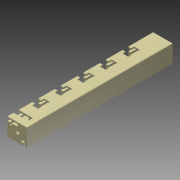
# Autodesk Inventor part: Pillar
Saved by Autodesk Inventor 2015 (Build 190159000, 159)
## iProperties
Created: 2015-04-20
Part Number: Pillar
Material: NylonD2W
Document SubType Name: Modeling
Designer: Akovo_000
Density: 1.13 g/cm^3
Appearance: Nylon 6
Mass: 42.2075 g
Surface Area: 197.531 cm^2
Volume: 37.3518 cm^3
Author: Akovo_000
Autodesk Inventor part; units mm, degrees
ref_plane "YZ Plane" through (0, 0, 0) normal (1, 0, 0) x (0, 1, 0)
ref_plane "XZ Plane" through (0, 0, 0) normal (0, 1, 0) x (-1, 0, 0)
ref_plane "XY Plane" through (0, 0, 0) normal (0, 0, 1) x (1, 0, 0)
sketch "Sketch1" plane through (0, 0, 0) normal (0, 1, 0) x (-1, 0, 0)
  line L0 (20, 18) -> (0, 18)
  line L1 (0, 18) -> (0, 0)
  line L2 (20, 18) -> (20, 16.5)
  line L3 (20, 16.5) -> (15.5, 16.5)
  line L4 (20, 14) -> (20, 0)
  line L5 (0, 0) -> (1.5, 0)
  line L6 (1.5, 0) -> (1.5, 4.5)
  line L7 (1.5, 4.5) -> (4, 4.5)
  line L8 (4, 0) -> (20, 0)
  circle A0 centre (10, 9) radius 2
  line L9 (15.5, 12) -> (17.5, 12)
  line L10 (17.5, 12) -> (17.5, 14)
  line L11 (17.5, 14) -> (20, 14)
  line L12 (15.5, 12) -> (15.5, 14)
  line L13 (4, 0) -> (4, 2.5)
  line L14 (4, 2.5) -> (6, 2.5)
  line L15 (6, 2.5) -> (6, 4.5)
  line L16 (4, 4.5) -> (6, 4.5)
  line L17 (10, 9) -> (0, 9) construction
  line L18 (10, 9) -> (20, 9) construction
  line L19 (10, 9) -> (10, 18) construction
  line L20 (10, 9) -> (10, 0) construction
  line L21 (15.5, 16.5) -> (9.5, 16.5)
  line L22 (9.5, 16.5) -> (9.5, 14)
  line L23 (15.5, 14) -> (9.5, 14)
  dimension "d0" = 2.5
  dimension "d2" = 20
  dimension "d3" = 1.5
  dimension "d7" = 4
  dimension "d13" = 2
  dimension "d26" = 18
  dimension "d84" = 4.5
  dimension "d85" = 4.5
  dimension "d86" = 6
  constraints: 48 end point, 8 equal length, 8 perpendicular, 7 horizontal, 5 point on line, 4 vertical, 2 collinear, 2 midpoint, 1 centre point, 1 parallel
  measures "d0" distance of L2.end L4.start
  measures "d2" distance between parallel lines of L1 L2
  measures "d3" distance between parallel lines of L3 L0
  measures "d7" diameter of A0
  measures "d13" distance of L9.start L12.end
  measures "d26" distance of L0.end L1.end
  measures "d84" distance of L5.end L6.end
  measures "d85" distance of L3.end L2.end
  measures "d86" distance of L21.end L3.end
extrude "Attachment Bas" add sketch "Sketch1" along normal blind 6.5
sketch "Sketch2" plane through (0, 6.5, 0) normal (0, 1, 0) x (1, 0, 0)
  circle A0 centre (-10, -9) radius 2 projected
  line L0 (-13.004, -6.2964) -> (-9.1606, -5.0467)
  line L1 (-9.1606, -5.0467) -> (-6.1566, -7.7503)
  line L2 (-6.1566, -7.7503) -> (-6.996, -11.7036)
  line L3 (-6.996, -11.7036) -> (-10.8394, -12.9533)
  line L4 (-10.8394, -12.9533) -> (-13.8434, -10.2497)
  line L5 (-13.8434, -10.2497) -> (-13.004, -6.2964)
  line L6 (-20, 0) -> (-13.004, -6.2964) construction
  line L7 (-13.004, -6.2964) -> (-10, -9) construction
  line L8 (0, -18) -> (-10, -9) construction
  dimension "d21" = 7
  constraints: 18 end point, 1 coincident, 1 collinear, 13 other
  measures "d21" distance between parallel lines of L1 L4
extrude "BossForNut" cut sketch "Sketch2" against normal blind 3.5
sketch "Sketch3" plane through (0, 6.5, 0) normal (0, 1, 0) x (1, 0, 0)
  line L0 (-1.5, 0) -> (0, 0)
  line L1 (0, 0) -> (-1.5, 0) projected
  line L2 (-4, 0) -> (-4, -2.5)
  line L3 (-4, -2.5) -> (-6, -2.5)
  line L4 (-6, -2.5) -> (-6, -4.5) projected
  line L5 (-6, -2.5) -> (-6, -4.5)
  line L6 (-6, -4.5) -> (-1.5, -4.5)
  line L7 (-6, -4.5) -> (-1.5, -4.5) projected
  line L8 (-1.5, -4.5) -> (-1.5, 0)
  line L9 (-1.5, 0) -> (-1.5, -4.5) projected
  line L10 (0, -18) -> (0, 0) construction
  line L11 (-20, -18) -> (-20, -16.5)
  line L12 (-20, -18) -> (-20, -16.5) projected
  line L13 (-20, -16.5) -> (-9.5, -16.5) projected
  line L14 (-15.5, -12) -> (-17.5, -12)
  line L15 (-15.5, -12) -> (-17.5, -12) projected
  line L16 (-17.5, -12) -> (-17.5, -14)
  line L17 (-17.5, -14) -> (-20, -14)
  line L18 (-17.5, -14) -> (-20, -14) projected
  line L19 (-6.1566, -7.7503) -> (-6.996, -11.7036) construction
  line L20 (-6.1566, -7.7503) -> (-9.1606, -5.0467)
  line L21 (-9.1606, -5.0467) -> (-6.1566, -7.7503) projected
  line L22 (-13.8434, -10.2497) -> (-10.8394, -12.9533)
  line L23 (-10.8394, -12.9533) -> (-13.8434, -10.2497) projected
  line L24 (-9.1606, -5.0467) -> (-14.768, 0)
  line L25 (-14.768, 0) -> (-4, 0)
  line L26 (-20, 0) -> (-4, 0) construction
  line L27 (-6.1566, -7.7503) -> (0, -13.2912)
  line L28 (0, -13.2912) -> (0, 0)
  line L29 (-10.8394, -12.9533) -> (-9.6764, -14)
  line L30 (0, -18) -> (-20, -18) construction
  line L31 (-5.232, -18) -> (-20, -18)
  line L32 (-20, -14) -> (-20, 0) construction
  line L33 (-13.8434, -10.2497) -> (-20, -4.7088)
  line L34 (-6.1566, -7.7503) -> (-6.996, -11.7036)
  line L35 (0, -18) -> (0, -13.2912)
  line L36 (-20, -4.7088) -> (-20, -14)
  line L37 (0, -18) -> (-5.232, -18)
  line L38 (-15.5, -12) -> (-15.5, -14)
  line L39 (-15.5, -14) -> (-15.5, -12) projected
  line L40 (-15.5, -14) -> (-9.5, -14)
  line L41 (-9.5, -14) -> (-9.5, -16.5)
  line L42 (-9.5, -16.5) -> (-20, -16.5)
  line L43 (-9.5, -14.1588) -> (-5.232, -18)
  line L44 (-9.5, -14.1588) -> (-9.6764, -14) construction
  line L45 (-6.996, -11.7036) -> (-10.8394, -12.9533)
  constraints: 60 end point, 21 collinear, 6 point on line, 4 perpendicular, 2 vertical
extrude "NutInserter" add sketch "Sketch3" along normal blind 5 contours L0 L28 L27 L20 L24 L25 L2 L3 L4 L6 L8 | L35 L37 L43 L41 L40 L29 L45 L34 L27 | L29 L40 L38 L14 L16 L17 L36 L33 L22
sketch "Sketch4" plane through (0, 11.5, 0) normal (0, 1, 0) x (1, 0, 0)
  line L0 (0, -17) -> (0, 0)
  line L1 (0, -18) -> (0, 0) projected
  line L2 (-15.5, -12) -> (-17.5, -12)
  line L3 (-17.5, -12) -> (-15.5, -12) projected
  line L4 (-17.5, -12) -> (-17.5, -14)
  line L5 (-17.5, -14) -> (-20, -14)
  line L6 (-4, 0) -> (-4, -2.5)
  line L7 (-4, -2.5) -> (-6, -2.5)
  line L8 (-6, -2.5) -> (-6, -4.5)
  line L9 (-6, -4.5) -> (-6, -2.5) projected
  line L10 (-6, -4.5) -> (-1.5, -4.5)
  line L11 (-1.5, -4.5) -> (-1.5, 0)
  line L12 (-1.5, 0) -> (0, 0)
  arc A0 (-1, -18) -> (0, -17) centre (-1, -17) ccw
  circle A1 centre (-10, -9) radius 2 projected
  line L13 (-20, -4.7088) -> (-20, -14) projected
  line L14 (-20, 0) -> (-15, -4.5) construction
  line L15 (-15, -4.5) -> (-10, -9) construction
  line L16 (-15, -4.5) -> (-13.3036, -9.717)
  line L17 (-12.8707, -11.0485) -> (-11.9109, -14)
  line L18 (-12.8707, -11.0485) -> (-13.3036, -9.717)
  line L19 (-14.9451, -10.608) -> (-12.8707, -11.0485)
  line L20 (-8.2093, -12.0382) -> (-6.1349, -12.4786)
  line L21 (-8.2093, -12.0382) -> (-12.8707, -11.0485)
  line L22 (-11.3971, -15.5801) -> (-9.975, -14) construction
  line L23 (-8.2093, -12.0382) -> (-6.7907, -10.4618)
  line L24 (-6.7907, -10.4618) -> (-3.6029, -6.9199)
  line L25 (-6.1349, -12.4786) -> (-6.7907, -10.4618)
  line L26 (-6.7907, -10.4618) -> (-8.2642, -5.9302)
  line L27 (-8.92, -3.9134) -> (-8.2642, -5.9302)
  line L28 (-3.6029, -6.9199) -> (-8.2642, -5.9302)
  line L29 (-8.2642, -5.9302) -> (-10.3387, -5.4897)
  line L30 (-10.3387, -5.4897) -> (-15, -4.5)
  line L31 (-8.92, -3.9134) -> (-10.3387, -5.4897)
  line L32 (-10.3387, -5.4897) -> (-13.5265, -9.0317)
  line L33 (-14.9451, -10.608) -> (-13.5265, -9.0317)
  line L34 (-6.1349, -12.4786) -> (-7.5, -11.25) construction
  line L35 (-4, 0) -> (-20, 0)
  line L36 (-4, 0) -> (-14.768, 0) projected
  line L37 (-20, 0) -> (-20, -14)
  line L38 (-20, -14) -> (-20, 0) projected
  line L39 (-1, -18) -> (-20, -18)
  line L40 (-20, -18) -> (-20, -16.5)
  line L41 (-20, -18) -> (-20, -16.5) projected
  line L42 (-20, -16.5) -> (-9.5, -16.5)
  line L43 (-20, -16.5) -> (-9.5, -16.5) projected
  line L44 (-9.5, -16.5) -> (-9.5, -14)
  line L45 (-9.5, -14) -> (-9.975, -14)
  line L46 (-9.975, -14) -> (-11.9109, -14)
  line L47 (-15.5, -14) -> (-15.5, -12)
  line L48 (-15.5, -12) -> (-15.5, -14) projected
  line L49 (-9.975, -14) -> (-8.2093, -12.0382)
  line L50 (-11.9109, -14) -> (-11.3971, -15.5801) construction
  line L51 (-11.9109, -14) -> (-15.5, -14)
  point P0 (-0.2929, -17.7071)
  dimension "d29" = 1
  dimension "d34" = 3.6029
  dimension "d37" = 2.6
  constraints: 86 end point, 21 collinear, 8 perpendicular, 6 point on line, 5 equal length, 3 point on circle, 2 tangent, 1 centre point, 1 coincident, 1 horizontal, 1 midpoint, 4 other
  measures "d29" radius of A0
  measures "d34" distance from line of L24.end L0
  measures "d37" distance from line of L21 L15.end
extrude "Main Pillar" add sketch "Sketch4" along normal blind 127
sketch "Sketch5" plane through (0, 138.5, 0) normal (0, 1, 0) x (1, 0, 0)
  line L0 (0, 0) -> (-1.5, 0)
  line L1 (-1.5, 0) -> (-1.5, -4.5)
  line L2 (-1.5, -4.5) -> (-1.5, 0) projected
  line L3 (-1.5, -4.5) -> (-6, -4.5)
  line L4 (-6, -4.5) -> (-1.5, -4.5) projected
  line L5 (-6, -4.5) -> (-6, -2.5)
  line L6 (-6, -2.5) -> (-6, -4.5) projected
  line L7 (-6, -2.5) -> (-4, -2.5)
  line L8 (-4, -2.5) -> (-6, -2.5) projected
  line L9 (-4, -2.5) -> (-4, 0)
  line L10 (-4, 0) -> (-4, -2.5) projected
  line L11 (-20, -14) -> (-17.5, -14)
  line L12 (-17.5, -14) -> (-20, -14) projected
  line L13 (-17.5, -14) -> (-17.5, -12)
  line L14 (-15.5, -12) -> (-17.5, -12) projected
  line L15 (-20, -18) -> (0, -18)
  line L16 (0, -18) -> (0, 0)
  line L17 (0, 0) -> (-1.5, 0) projected
  circle A0 centre (-10, -9) radius 2 projected
  line L18 (-13.8434, -10.2497) -> (-10.8394, -12.9533)
  line L19 (-10.8394, -12.9533) -> (-13.8434, -10.2497) projected
  line L20 (-10.8394, -12.9533) -> (-6.996, -11.7036)
  line L21 (-6.1566, -7.7503) -> (-9.1606, -5.0467)
  line L22 (-9.1606, -5.0467) -> (-6.1566, -7.7503) projected
  line L23 (-4, 0) -> (-14.768, 0)
  line L24 (-4, 0) -> (-20, 0) construction
  line L25 (-14.768, 0) -> (-9.1606, -5.0467)
  line L26 (-13.8434, -10.2497) -> (-20, -4.7088)
  line L27 (-20, -14) -> (-20, -4.7088)
  line L28 (-20, -18) -> (-20, -16.5)
  line L29 (-9.5, -16.5) -> (-9.5, -14)
  line L30 (-9.5, -16.5) -> (-9.5, -14) projected
  line L31 (-9.5, -14) -> (-15.5, -14)
  line L32 (-9.5, -14) -> (-15.5, -14) projected
  line L33 (-15.5, -12) -> (-17.5, -12)
  line L34 (-20, -16.5) -> (-9.5, -16.5)
  line L35 (-15.5, -12) -> (-15.5, -14)
  line L36 (-15.5, -12) -> (-15.5, -14) projected
  line L37 (-6.1566, -7.7503) -> (-6.996, -11.7036)
  constraints: 48 end point, 14 collinear, 2 horizontal, 2 perpendicular, 1 coincident, 1 point on line, 1 vertical
extrude "NutInserter2" add sketch "Sketch5" along normal blind 5 contours L16 L15 L28 L34 L29 L31 L35 L14 L13 L11 L27 L26 L18 L20 L37 L21 L25 L23 L9 L7 L5 L3 L1 L0
sketch "Sketch6" plane through (0, 143.5, 0) normal (0, 1, 0) x (1, 0, 0)
  line L0 (-4, 0) -> (-4, -2.5)
  line L1 (-4, -2.5) -> (-6, -2.5)
  line L2 (-4, -2.5) -> (-6, -2.5) projected
  line L3 (-6, -2.5) -> (-6, -4.5)
  line L4 (-6, -2.5) -> (-6, -4.5) projected
  line L5 (-6, -4.5) -> (-1.5, -4.5)
  line L6 (-6, -4.5) -> (-1.5, -4.5) projected
  line L7 (-1.5, -4.5) -> (-1.5, 0)
  line L8 (-1.5, 0) -> (0, 0)
  line L9 (-1.5, 0) -> (0, 0) projected
  line L10 (0, 0) -> (0, -18)
  line L11 (0, -18) -> (-20, -18)
  line L12 (-20, 0) -> (-20, -4.7088) projected
  line L13 (-4, 0) -> (-20, 0)
  line L14 (-13.8434, -10.2497) -> (-13.004, -6.2964)
  line L15 (-13.8434, -10.2497) -> (-13.004, -6.2964) projected
  line L16 (-13.004, -6.2964) -> (-9.1606, -5.0467)
  line L17 (-13.004, -6.2964) -> (-9.1606, -5.0467) projected
  line L18 (-6.1566, -7.7503) -> (-9.1606, -5.0467)
  line L19 (-9.1606, -5.0467) -> (-6.1566, -7.7503) projected
  line L20 (-6.1566, -7.7503) -> (-6.996, -11.7036)
  line L21 (-6.1566, -7.7503) -> (-6.996, -11.7036) projected
  line L22 (-6.996, -11.7036) -> (-10.8394, -12.9533)
  line L23 (-6.996, -11.7036) -> (-10.8394, -12.9533) projected
  line L24 (-10.8394, -12.9533) -> (-13.8434, -10.2497)
  line L25 (-10.8394, -12.9533) -> (-13.8434, -10.2497) projected
  line L26 (-20, 0) -> (-20, -14)
  line L27 (-20, -14) -> (-17.5, -14)
  line L28 (-17.5, -14) -> (-17.5, -12)
  line L29 (-17.5, -12) -> (-17.5, -14) projected
  line L30 (-17.5, -12) -> (-15.5, -12)
  line L31 (-15.5, -12) -> (-15.5, -14)
  line L32 (-15.5, -14) -> (-15.5, -12) projected
  line L33 (-15.5, -14) -> (-9.5, -14)
  line L34 (-9.5, -14) -> (-15.5, -14) projected
  line L35 (-9.5, -14) -> (-9.5, -16.5)
  line L36 (-9.5, -16.5) -> (-9.5, -14) projected
  line L37 (-9.5, -16.5) -> (-20, -16.5)
  line L38 (-20, -16.5) -> (-20, -18)
  circle A0 centre (-10, -9) radius 2 projected
  line L39 (-10, -9) -> (-10.8394, -12.9533) construction
  line L40 (-10, -9) -> (-9.1606, -5.0467) construction
  constraints: 52 end point, 15 collinear, 7 perpendicular, 1 vertical
extrude "BossFotNut2" add sketch "Sketch6" along normal blind 3.5 contours L0 L1 L3 L5 L7 L8 L10 L11 L38 L37 L35 L33 L31 L30 L28 L27 L26 L12 L13
sketch "Sketch7" plane through (0, 147, 0) normal (0, 1, 0) x (1, 0, 0)
  line L0 (0, 0) -> (0, -18)
  line L1 (0, -18) -> (-20, -18)
  line L2 (-20, 0) -> (-4, 0)
  line L3 (-4, 0) -> (-4, -2.5)
  line L4 (-4, -2.5) -> (-4, 0) projected
  line L5 (-4, -2.5) -> (-6, -2.5)
  line L6 (-6, -2.5) -> (-6, -4.5)
  line L7 (-6, -4.5) -> (-1.5, -4.5)
  line L8 (0, 0) -> (-1.5, 0)
  line L9 (-1.5, -4.5) -> (-6, -4.5) projected
  line L10 (-1.5, 0) -> (-1.5, -4.5)
  line L11 (0, 0) -> (-1.5, 0) projected
  circle A0 centre (-10, -9) radius 2 projected
  line L12 (-20, -18) -> (-20, -16.5)
  line L13 (-20, -16.5) -> (-20, -18) projected
  line L14 (-9.5, -16.5) -> (-9.5, -14)
  line L15 (-9.5, -14) -> (-15.5, -14)
  line L16 (-15.5, -14) -> (-9.5, -14) projected
  line L17 (-15.5, -14) -> (-15.5, -12)
  line L18 (-15.5, -12) -> (-15.5, -14) projected
  line L19 (-15.5, -12) -> (-17.5, -12)
  line L20 (-17.5, -12) -> (-17.5, -14)
  line L21 (-17.5, -14) -> (-17.5, -12) projected
  line L22 (-17.5, -14) -> (-20, -14)
  line L23 (-20, -14) -> (-17.5, -14) projected
  line L24 (-20, -14) -> (-20, 0)
  line L25 (-20, 0) -> (-20, -14) projected
  line L26 (-20, -16.5) -> (-9.5, -16.5)
  constraints: 36 end point, 7 collinear, 6 perpendicular, 2 horizontal, 2 vertical
extrude "Attachment Base 2" add sketch "Sketch7" along normal blind 3
sketch "ShelvStack" plane through (-4, 0, 0) normal (0, 0, -1) x (-1, 0, 0)
  line L0 (16, 138.5) -> (6.95, 138.5)
  line L1 (6.95, 138.5) -> (6.95, 127.4167)
  line L2 (16, 93.1) -> (16, 138.5)
  line L3 (16, 104.2333) -> (16, 115.3167)
  line L4 (6.95, 104.2333) -> (6.95, 92.1333)
  line L5 (6.95, 57.8667) -> (6.95, 45.7667)
  line L6 (16, 45.7667) -> (16, 34.6833)
  line L7 (6.95, 34.6833) -> (6.95, 22.5833)
  line L8 (16, 11.5) -> (6.95, 11.5)
  line L9 (6.95, 11.5) -> (6.95, 22.5833)
  line L10 (16, 22.5833) -> (16, 11.5)
  line L11 (6.95, 115.3167) -> (12.95, 115.3167)
  line L12 (12.95, 127.4167) -> (6.95, 127.4167)
  line L13 (6.95, 127.4167) -> (6.95, 115.3167)
  line L14 (16, 127.4167) -> (16, 124.3667)
  line L15 (12.95, 124.3667) -> (12.95, 127.4167)
  line L16 (12.95, 124.3667) -> (16, 124.3667)
  line L17 (12.95, 115.3167) -> (12.95, 118.3667)
  line L18 (12.95, 118.3667) -> (16, 118.3667)
  line L19 (16, 118.3667) -> (16, 115.3167)
  line L20 (6.95, 92.1333) -> (12.95, 92.1333)
  line L21 (12.95, 104.2333) -> (6.95, 104.2333)
  line L22 (6.95, 104.2333) -> (6.95, 92.1333)
  line L23 (16, 104.2333) -> (16, 101.1833)
  line L24 (12.95, 101.1833) -> (12.95, 104.2333)
  line L25 (12.95, 101.1833) -> (16, 101.1833)
  line L26 (12.95, 92.1333) -> (12.95, 95.1833)
  line L27 (12.95, 95.1833) -> (16, 95.1833)
  line L28 (16, 92.1333) -> (16, 95.1833)
  line L29 (6.95, 45.7667) -> (12.95, 45.7667)
  line L30 (12.95, 57.8667) -> (6.95, 57.8667)
  line L31 (6.95, 57.8667) -> (6.95, 45.7667)
  line L32 (12.95, 57.8667) -> (12.95, 54.8167)
  line L33 (12.95, 54.8167) -> (16, 54.8167)
  line L34 (16, 54.8167) -> (16, 57.8667)
  line L35 (16, 54.8167) -> (16, 57.8667)
  line L36 (16, 45.7667) -> (16, 48.8167)
  line L37 (16, 48.8167) -> (12.95, 48.8167)
  line L38 (12.95, 48.8167) -> (12.95, 45.7667)
  line L39 (6.95, 22.5833) -> (12.95, 22.5833)
  line L40 (12.95, 34.6833) -> (6.95, 34.6833)
  line L41 (6.95, 34.6833) -> (6.95, 22.5833)
  line L42 (12.95, 22.5833) -> (12.95, 25.6333)
  line L43 (12.95, 25.6333) -> (16, 25.6333)
  line L44 (16, 22.5833) -> (16, 25.6333)
  line L45 (12.95, 34.6833) -> (12.95, 31.6333)
  line L46 (12.95, 31.6333) -> (16, 31.6333)
  line L47 (16, 31.6333) -> (16, 34.6833)
  line L48 (16, 124.3667) -> (16, 118.3667)
  line L49 (16, 101.1833) -> (16, 95.1833)
  line L50 (16, 54.8167) -> (16, 48.8167)
  line L51 (16, 31.6333) -> (16, 25.6333)
  line L52 (6.95, 127.4167) -> (6.95, 115.3167)
  line L53 (6.95, 34.6833) -> (6.95, 45.7667)
  line L54 (6.95, 104.2333) -> (6.95, 115.3167)
  line L55 (6.95, 22.5833) -> (6.95, 22.5833)
  line L56 (12.95, 22.5833) -> (16, 22.5833)
  line L57 (16, 34.6833) -> (12.95, 34.6833)
  line L58 (6.95, 34.6833) -> (6.95, 34.6833)
  line L59 (6.95, 45.7667) -> (6.95, 45.7667)
  line L60 (12.95, 45.7667) -> (16, 45.7667)
  line L61 (12.95, 57.8667) -> (16, 57.8667)
  line L62 (6.95, 57.8667) -> (6.95, 57.8667)
  line L63 (6.95, 92.1333) -> (6.95, 92.1333)
  line L64 (12.95, 92.1333) -> (16, 92.1333)
  line L65 (12.95, 104.2333) -> (16, 104.2333)
  line L66 (6.95, 104.2333) -> (6.95, 104.2333)
  line L67 (12.95, 115.3167) -> (16, 115.3167)
  line L68 (6.95, 115.3167) -> (6.95, 115.3167)
  line L69 (6.95, 127.4167) -> (6.95, 127.4167)
  line L70 (12.95, 127.4167) -> (16, 127.4167)
  line L71 (16, 0) -> (0, 0) projected
  line L72 (6.95, 92.1333) -> (6.95, 81.05)
  line L73 (6.95, 81.05) -> (6.95, 68.95)
  line L74 (6.95, 68.95) -> (6.95, 57.8667)
  line L75 (6.95, 81.05) -> (12.95, 81.05)
  line L76 (16, 11.5) -> (16, 138.5) construction
  line L77 (6.95, 68.95) -> (12.95, 68.95)
  line L78 (12.95, 81.05) -> (12.95, 78)
  line L79 (12.95, 78) -> (16, 78)
  line L80 (12.95, 68.95) -> (12.95, 72)
  line L81 (12.95, 72) -> (16, 72)
  line L82 (16, 72) -> (16, 68.95)
  line L83 (16, 78) -> (16, 81.05)
  line L84 (16, 92.1333) -> (16, 81.05)
  line L85 (16, 68.95) -> (16, 57.8667)
  line L86 (16, 78) -> (16, 72)
  line L87 (0, 150) -> (16, 150) projected
  line L88 (12.95, 81.05) -> (16, 81.05)
  line L89 (12.95, 68.95) -> (16, 68.95)
  dimension "d57" = 6
  dimension "d58" = 12.1
  dimension "d60" = 6
  dimension "d87" = 150
  constraints: 174 end point, 42 equal length, 25 collinear, 14 parallel, 12 perpendicular, 12 vertical, 7 horizontal, 7 point on line
  measures "d57" distance between parallel lines of L18 L16
  measures "d58" distance between parallel lines of L12 L11
  measures "d60" distance of L12.end L12.start
  measures "d87" distance between parallel lines of L71 L87
extrude "Extrusion11" cut sketch "ShelvStack" against normal blind 25 contours L12 L15 L16 L2 L18 L17 L11 L13 | L21 L24 L25 L2 L27 L26 L20 L4 | L75 L78 L79 L86 L81 L80 L77 L73 | L30 L32 L33 L50 L37 L38 L29 L5 | L40 L45 L46 L51 L43 L42 L39 L7
body "Solid1"
